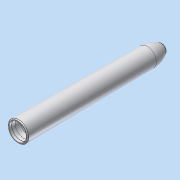
# Autodesk Inventor part: Body
Saved by Autodesk Inventor 2012 (Build 160160000, 160)
## iProperties
Created: 2015-03-22
Part Number: Body
Material: Default
Document SubType Name: Modeling
Designer: Jason
Density: 1 g/cm^3
Author: Jason
Autodesk Inventor part; units mm, degrees
ref_plane "YZ Plane" through (0, 0, 0) normal (1, 0, 0) x (0, 1, 0)
ref_plane "XZ Plane" through (0, 0, 0) normal (0, 1, 0) x (-1, 0, 0)
ref_plane "XY Plane" through (0, 0, 0) normal (0, 0, 1) x (1, 0, 0)
sketch "Revolution Sketch" plane through (0, 0, 0) normal (1, 0, 0) x (0, 1, 0)
  line L0 (5.55, 0) -> (-5.55, 0) construction
  arc A0 (6.05, -0.5) -> (5.55, 0) centre (5.55, -0.5) ccw
  line L1 (6.05, -0.5) -> (6.15, -0.5)
  line L2 (6.15, -0.5) -> (5.5, -77.26)
  line L3 (5.5, -77.26) -> (0, -77.26) construction
  arc A1 (3.05, -85.46) -> (5.5, -77.26) centre (-9.8834, -77.1297) ccw
  line L4 (3.05, -85.46) -> (3, -85.46)
  arc A2 (1.4584, -85.76) -> (3, -85.46) centre (2.2, -85.46) ccw construction
  line L5 (1.4584, -85.76) -> (0.1, -85.76) construction
  line L6 (0.1, -85.76) -> (0, -85.86)
  line L7 (5.55, 0) -> (0, 0)
  line L8 (3, -85.46) -> (3, -86.26) construction
  line L9 (3, -86.26) -> (0, -86.26) construction
  line L10 (0, -86.26) -> (0, -85.86) construction
  line L11 (1, -85.76) -> (1.846, -86.1774)
  arc A3 (1.846, -86.1774) -> (3, -85.46) centre (2.2, -85.46) ccw construction
  line L12 (1, -85.76) -> (0.1, -85.76)
  line L13 (6.05, -0.5) -> (6.05, 0) construction
  line L14 (5.55, 0) -> (6.05, 0)
  line L15 (1, -85.76) -> (1, -86.26) construction
  line L16 (0, -85.86) -> (0, 0)
  line L17 (0, -103.8185) -> (0, 17.4239) projected
  arc A4 (2.4982, -86.26) -> (5.5, -77.26) centre (-9.8834, -77.1297) ccw construction
  arc A5 (2.7181, -85.954) -> (3, -85.46) centre (0.1927, -84.1856) ccw
  arc A6 (1.846, -86.1774) -> (2.7181, -85.954) centre (2.1519, -85.5575) ccw
  point P0 (0, -86.06)
  dimension "d0" = 6.15
  dimension "d1" = 5.5
  dimension "d2" = 86.26
  dimension "d3" = 0.1
  dimension "d4" = 0.5
  dimension "d5" = 9
  dimension "d6" = 0.05
  dimension "d8" = 0.5
  dimension "d9" = 1
  dimension "d10" = 3
  dimension "d11" = 0.8
  dimension "d12" = 0.1
  dimension "d13" = 0.1
  constraints: 34 end point, 16 point on circle, 14 tangent, 9 horizontal, 7 centre point, 5 vertical, 3 point on line, 2 coincident, 2 midpoint, 2 vertical alignment, 1 concentric
  measures "d0" horizontal distance of point (0, 0) L1.end
  measures "d1" horizontal distance of point (0, 0) L2.end
  measures "d2" distance between parallel lines of L9 L0
  measures "d3" distance of L1.start L1.end
  measures "d4" radius of A0
  measures "d5" distance between parallel lines of L9 L3
  measures "d6" distance of L4.start L4.end
  measures "d8" distance between parallel lines of L9 L5
  measures "d9" distance between parallel lines of L10 L15
  measures "d10" distance from line of L10 L4.end
  measures "d11" radius of A2
  measures "d12" distance from line of L16 L5.end
  measures "d13" horizontal distance of L5.end L6.end
revolve "Revolution" add sketch "Revolution Sketch" angle 360 about axis through (0, 0, -10) along (0, 0, 1)
sketch "Sketch3" plane through (0, 0, 0) normal (1, 0, 0) x (0, 1, 0)
  line L0 (5.15, 2) -> (5.15, -1.5)
  line L1 (5.15, -1.5) -> (5.05, -1.5)
  line L2 (5.05, -1.5) -> (5.05, -3.5)
  line L3 (5.05, -3.5) -> (5.15, -3.5)
  line L4 (5.15, -3.5) -> (5.15, -6.5)
  line L5 (5.15, -6.5) -> (5.05, -6.5)
  line L6 (5.05, -6.5) -> (5.05, -8)
  line L7 (5.05, -8) -> (5.15, -8)
  line L8 (5.15, -8) -> (5.15, -77.2454)
  arc A0 (3.05, -85.46) -> (5.5, -77.26) centre (-9.8834, -77.1297) ccw projected
  arc A1 (3.0702, -84.76) -> (5.15, -77.2454) centre (-9.8834, -77.1297) ccw
  line L9 (3.0702, -84.76) -> (0, -84.76)
  line L10 (-1, -85.76) -> (1, -85.76) construction
  line L11 (-5.55, 0) -> (5.55, 0) construction
  line L12 (5.15, 2) -> (0, 2)
  line L13 (0, 2) -> (0, -84.76)
  point P0 (0, 0)
  point P1 (0, -41.38)
  point P2 (0, 0)
  dimension "d16" = 1
  dimension "d17" = 5.15
  dimension "d18" = 0.1
  dimension "d19" = 1.5
  dimension "d20" = 2
  dimension "d21" = 3
  dimension "d22" = 1.5
  dimension "d23" = 0.3501
  dimension "d24" = 2
  constraints: 24 end point, 6 horizontal, 6 vertical, 3 collinear, 2 midpoint, 2 point on circle, 1 centre point, 1 vertical alignment
  measures "d16" distance between parallel lines of L10 L9
  measures "d17" distance from line of L0 point (0, 0)
  measures "d18" distance between parallel lines of L0 L2
  measures "d19" distance between parallel lines of L11 L1
  measures "d20" distance of L1.end L2.end
  measures "d21" distance between parallel lines of L5 L3
  measures "d22" distance between parallel lines of L7 L5
  measures "d23" radial gap between concentric circles of A1 A0
  measures "d24" distance between parallel lines of L11 L12
revolve "Revolution2" cut sketch "Sketch3" angle 360 about axis through (0, 0, 2) along (0, 0, -1)
sketch "Sketch4" plane through (0, 0, 0) normal (1, 0, 0) x (0, 1, 0)
  arc A0 (3.0702, -84.76) -> (5.15, -77.2454) centre (-9.8834, -77.1297) ccw projected
  line L0 (3.0702, -84.76) -> (-3.0702, -84.76) construction
  line L1 (3.0702, -84.76) -> (2, -84.76)
  line L2 (5.15, -8) -> (5.15, -77.2454) construction
  line L3 (5.15, -77.2454) -> (5.15, -66.76)
  line L4 (5.15, -66.76) -> (2, -66.76)
  line L5 (2, -66.76) -> (2, -84.76)
  point P0 (0, 0)
  point P1 (5.15, -72.0273)
  dimension "d26" = 18
  dimension "d27" = 2
  constraints: 8 end point, 2 horizontal, 2 point on line, 1 vertical
  measures "d26" distance between parallel lines of L0 L4
  measures "d27" distance from line of point (0, 0) L5
extrude "Extrusion1" add sketch "Sketch4" along normal mid plane 0.1
pattern_circular "Circular Pattern1" count 6 over 360 about axis through (0, 0, -10) along (0, 0, 1) of "Extrusion1"
chamfer "Chamfer1" distance 1.5 angle 45 6 edges at (0, 2, -66.76) (1.7321, 1, -66.76) (1.7321, -1, -66.76) (-1.7321, 1, -66.76) (-1.7321, -1, -66.76) (0, -2, -66.76)
equation "\"d22\" = d19"
equation "\"d12\" = d13"
body "Solid1"
